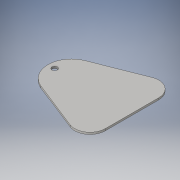
# Autodesk Inventor part: Layla_Top
Saved by Autodesk Inventor 2016 (Build 200138000, 138)
## iProperties
Created: 2016-07-06
Part Number: Layla_Top
Material: Generic
Document SubType Name: Modeling
Designer: Ryker
Density: 1 g/cm^3
Appearance: Default
Author: Ryker
Autodesk Inventor part; units mm, degrees
ref_plane "YZ Plane" through (0, 0, 0) normal (1, 0, 0) x (0, 1, 0)
ref_plane "XZ Plane" through (0, 0, 0) normal (0, 1, 0) x (-1, 0, 0)
ref_plane "XY Plane" through (0, 0, 0) normal (0, 0, 1) x (1, 0, 0)
sketch "Sketch1" plane through (0, 0, 0) normal (0, 1, 0) x (-1, 0, 0)
  arc A0 (-401.8239, -177.8) -> (-262.982, -272.3283) centre (-300.2239, -177.8) ccw
  arc A1 (-262.982, 272.3283) -> (-401.8239, 177.8) centre (-300.2239, 177.8) ccw
  arc A2 (57.5403, -146.05) -> (57.5403, 146.05) centre (0, 0) ccw
  line L0 (57.5403, -146.05) -> (-262.982, -272.3283)
  line L1 (57.5403, 146.05) -> (-262.982, 272.3283)
  line L2 (-401.8239, 177.8) -> (-401.8239, -177.8)
  circle A3 centre (112.5261, 0) radius 18.2417
  point P0 (0, 0)
  point P1 (156.9761, 0)
  dimension "d14" = 292.1
  dimension "d15" = 355.6
  dimension "d17" = 101.6
  dimension "d18" = 156.9761
  dimension "d20" = 36.4834
  dimension "d21" = 44.45
  dimension "d22" = 558.8
  dimension "d29" = 156.9761
  dimension "d30" = 115.7292
  constraints: 7 point on circle, 6 end point, 6 tangent, 4 centre point, 1 equal radius, 1 vertical, 1 vertical alignment
  measures "d14" distance of L1.start L0.start
  measures "d15" distance of L2.start L2.end
  measures "d17" radius of A1
  measures "d18" radius of A2
  measures "d20" diameter of A3
  measures "d21" distance of point (156.976, 0) A3.centre
  measures "d22" distance from line of L2 point (156.976, 0)
  measures "d29" distance from line of point (0, 0) L0
  measures "d30" distance from line of A3.centre L0
extrude "Extrusion1" add sketch "Sketch1" along normal blind 12.7
body "Solid1"
